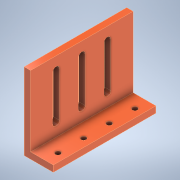
# Autodesk Inventor part: pullyBracketLowerPortion
Saved by Autodesk Inventor 2022.1 (Build 261234020, 234B)
## iProperties
Created: 2021-11-10
Part Number: pullyBracketLowerPortion
Material: PC/ABS Plastic
Document SubType Name: Modeling
Designer: robst
Density: 0.357273 g/cm^3
Appearance: Smooth - Light Orange
Author: robst
Autodesk Inventor part; units mm, degrees
ref_plane "YZ Plane" through (0, 0, 0) normal (1, 0, 0) x (0, 1, 0)
ref_plane "XZ Plane" through (0, 0, 0) normal (0, 1, 0) x (-1, 0, 0)
sketch "Sketch1" plane through (0, 0, 0) normal (0, 1, 0) x (-1, 0, 0)
  line L0 (11.2547, 50.8) -> (-11.2547, 50.8)
  line L1 (-11.2547, 50.8) -> (-11.2547, -50.8)
  line L2 (-11.2547, -50.8) -> (11.2547, -50.8)
  line L3 (11.2547, -50.8) -> (11.2547, 50.8)
  line L4 (11.2547, 50.8) -> (-11.2547, -50.8) construction
  line L5 (-11.2547, 50.8) -> (11.2547, -50.8) construction
  point P0 (0, 0)
  dimension "d0" = 101.6
  dimension "d1" = 22.5095
  constraints: 12 end point, 2 midpoint, 2 parallel, 1 horizontal, 1 perpendicular
  measures "d0" distance of L2.end L0.start
  measures "d1" distance of L1.end L2.end
extrude "Extrusion1" add sketch "Sketch1" against normal blind 6.35
sketch "Sketch2" plane through (0, 0, 0) normal (0, 1, 0) x (1, 0, 0)
  line L0 (11.2547, -50.8) -> (-11.2547, -50.8) projected
  line L1 (-11.2547, 50.8) -> (11.2547, 50.8) projected
  line L2 (-11.2547, -50.8) -> (-4.9047, -50.8)
  line L3 (-4.9047, -50.8) -> (-4.9047, 50.8)
  line L4 (-4.9047, 50.8) -> (-11.2547, 50.8)
  line L5 (-11.2547, 50.8) -> (-11.2547, -50.8)
  point P0 (0, 0)
  dimension "d4" = 6.35
  constraints: 8 end point, 2 parallel, 1 horizontal, 1 perpendicular, 1 point on line
  measures "d4" distance between parallel lines of L3 L5
extrude "Extrusion2" add sketch "Sketch2" along normal blind 76.2
sketch "Sketch4" plane through (0, 0, 0) normal (0, 1, 0) x (1, 0, 0)
  line L0 (-4.9047, -50.8) -> (11.2547, -50.8) construction
  line L1 (3.175, -50.8) -> (3.175, 50.8) construction
  line L2 (-11.2547, 50.8) -> (11.2547, 50.8) construction
  point P0 (0, 0)
  point P1 (3.175, -38.1)
  point P2 (3.175, -12.7)
  point P3 (3.175, 12.7)
  point P4 (3.175, 38.1)
  dimension "d11" = 12.7
  dimension "d14" = 25.4
  constraints: 2 end point, 2 point on line, 2 vertical, 1 midpoint, 3 other
  measures "d11" distance from line of point (3.175, -38.1) L0
  measures "d14" distance of point (3.175, -38.1) point (3.175, -12.7)
hole "Hole1" at (3.175, 0, 38.1) at (3.175, 0, 12.7) at (3.175, 0, -12.7) at (3.175, 0, -38.1) direction (0, -1, 0) diameter 5.1054 end through all clearance for "Hex Machine Screw" size "#10" standard "Ansi Unified Screw Threads"
ref_plane "Work Plane1" through (-11.2547, -6.35, -50.8) normal (-1, 0, 0) x (0, 0, 1)
sketch "Sketch7" plane through (-11.2547, -6.35, -50.8) normal (-1, 0, 0) x (0, 0, 1)
  line L0 (0, 6.35) -> (101.6, 6.35) projected
  line L1 (0, 82.55) -> (101.6, 82.55) projected
  line L2 (101.6, 0) -> (101.6, 82.55) projected
  line L3 (0, 0) -> (0, 82.55) projected
  line L4 (101.6, 6.35) -> (101.6, 82.55) projected
  line L5 (0, 6.35) -> (101.6, 6.35)
  line L6 (101.6, 6.35) -> (101.6, 82.55)
  line L7 (101.6, 82.55) -> (0, 82.55)
  line L8 (0, 82.55) -> (0, 6.35)
  point P0 (50.8, 6.35)
  constraints: 8 end point, 2 parallel, 1 horizontal, 1 perpendicular
extrude "Extrusion5" cut sketch "Sketch7" against normal through all
sketch "Sketch8" plane through (-11.2547, -6.35, -50.8) normal (-1, 0, 0) x (0, 0, 1)
  line L0 (0, 0) -> (0, 6.35) projected
  line L1 (101.6, 0) -> (101.6, 6.35) projected
  line L2 (101.6, 0) -> (0, 0) projected
  line L3 (0, 0) -> (101.6, 0)
  line L4 (101.6, 0) -> (101.6, 76.2)
  line L5 (101.6, 76.2) -> (0, 76.2)
  line L6 (0, 76.2) -> (0, 0)
  point P0 (50.8, 6.35)
  dimension "d51" = 76.2
  constraints: 8 end point, 2 parallel, 1 horizontal, 1 perpendicular
  measures "d51" distance between parallel lines of L5 L2
extrude "Extrusion6" add sketch "Sketch8" along normal blind 6.35
sketch "Sketch9" plane through (-11.2547, -6.35, -50.8) normal (1, 0, 0) x (0, 0, -1)
  line L0 (-101.6, 76.2) -> (0, 76.2) projected
  line L1 (0, 76.2) -> (0, 0) projected
  line L2 (-101.6, 0) -> (-101.6, 76.2) projected
  line L3 (0, 0) -> (-101.6, 0) projected
  line L4 (-76.2, 63.5) -> (-76.2, 19.05) construction
  line L5 (-79.5782, 63.5) -> (-79.5782, 19.05)
  line L6 (-72.8218, 19.05) -> (-72.8218, 63.5)
  arc A0 (-72.8218, 63.5) -> (-79.5782, 63.5) centre (-76.2, 63.5) ccw
  arc A1 (-79.5782, 19.05) -> (-72.8218, 19.05) centre (-76.2, 19.05) ccw
  line L7 (-101.6, 63.5) -> (0, 63.5) construction
  line L8 (-101.6, 19.05) -> (0, 19.05) construction
  line L9 (-50.8, 63.5) -> (-50.8, 19.05) construction
  line L10 (-54.1782, 63.5) -> (-54.1782, 19.05)
  line L11 (-47.4218, 19.05) -> (-47.4218, 63.5)
  arc A2 (-47.4218, 63.5) -> (-54.1782, 63.5) centre (-50.8, 63.5) ccw
  arc A3 (-54.1782, 19.05) -> (-47.4218, 19.05) centre (-50.8, 19.05) ccw
  line L12 (-25.4, 63.5) -> (-25.4, 19.05) construction
  line L13 (-28.7782, 63.5) -> (-28.7782, 19.05)
  line L14 (-22.0218, 19.05) -> (-22.0218, 63.5)
  arc A4 (-22.0218, 63.5) -> (-28.7782, 63.5) centre (-25.4, 63.5) ccw
  arc A5 (-28.7782, 19.05) -> (-22.0218, 19.05) centre (-25.4, 19.05) ccw
  point P0 (-50.8, 6.35)
  point P1 (-76.2, 41.275)
  point P2 (-50.8, 41.275)
  point P3 (-25.4, 41.275)
  dimension "d54" = 25.4
  dimension "d55" = 12.7
  dimension "d56" = 19.05
  dimension "d58" = 6.7564
  dimension "d59" = 25.4
  constraints: 28 end point, 12 point on circle, 12 tangent, 6 centre point, 6 point on line, 5 midpoint, 3 parallel, 3 perpendicular, 2 equal radius, 1 vertical
  measures "d54" distance between parallel lines of L4 L2
  measures "d55" distance from line of L4.start L0
  measures "d56" distance from line of L3 L4.end
  measures "d58" distance between parallel lines of L6 L5
  measures "d59" distance between parallel lines of L9 L12
extrude "Extrusion7" cut sketch "Sketch9" against normal through all contours A0 L6 A1 L5 | A2 L11 A3 L10 | A4 L14 A5 L13
equation "\"d0\" = BaseLength"
equation "\"d1\" = BaseWidth"
equation "\"d2\" = BaseThickness"
equation "\"d4\" = BackWidth"
equation "\"d5\" = BackHeight"
equation "\"d11\" = offsetForFirstHole"
equation "\"d54\" = deltaForSlots"
equation "\"BaseWidth\" = 22.50948"
equation "\"BaseLength\" = 101.6"
equation "\"BaseThickness\" = 6.35"
equation "\"BackWidth\" = 6.35"
equation "\"BackHeight\" = 76.2"
equation "\"TopBackExtension\" = 50.8"
equation "\"TopFrontExtension\" = 50.8"
equation "\"TopThickness\" = 6.35"
equation "\"offsetForFirstHole\" = 12.7"
equation "\"holeSpacingForMotorBracket\" = 76.2"
equation "\"offsetForBracketHoleFromEdge\" = 6.35"
equation "\"holeSpacingForVariationInMotorBracketHoles\" = 19.05"
equation "\"deltaForSlots\" = 0.25 * BaseLength"
body "Solid1"
